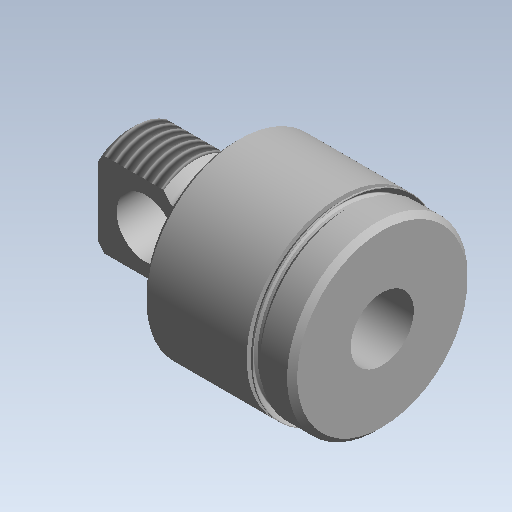
# Autodesk Inventor part: 09P0Y000_rear_head
Saved by Autodesk Inventor 2020 (Build 240168000, 168)
## iProperties
Part Number: 09P0Y000_rear_head
Material: Generic
Catalog Web Link: www.cadenas.de
Description: Rear Head-Original Line - Standard Air Cylinders
Vendor: BIMBA
Document SubType Name: Modeling
Designer: partserver
Manufacturer: BIMBA
Mass: 12.8782 g
Surface Area: 50.1592 cm^2
Volume: 12.8782 cm^3
Density: 1 g/cm^3
Appearance: PSOLRGB-211-211-211
Category: PARTsolutions
Company: BIMBA
PSOL_IDENT_0: {$CADENAS_DATA\23d-libs\bimba\bimba_brand\bimba_imperial\bimba_full_line\original_line_cylinders\sta
PSOL_IDENT_1: ndard_air_cylinders\rear_head.prj},241 {VTYP=3D},{NB=09P0Y000_rear_head},{LINA=09P0Y000_rear_head},{
PSOL_IDENT_2: NN=Rear Head},{DATE=19.01.2022 10:19:37},{GEOMDATE=11.01.2022 11:41:00},{VERSION=},{LINEID=60},{WBVA
PSOL_IDENT_3: R=MNT,ACTING,DER,Q,T1,T2,T3,T4,TRIM,Y,K,MB,CUSH,FBON},{WBNUMERIC=TRIM,MB,CUSH}  {NB=09P0Y000_rear_he
PSOL_IDENT_4: ad},{LINA=09P0Y000_rear_head},{KT=DUMMY},{PN=09P0Y000},{BORE=1.06250},{BOREPN=09},{MNT=P},{MNTALG=''
PSOL_IDENT_5: , 'Front Nose' , 'P' , 'Rear Pivot' , 'S' , 'Built-in Valve S' , 'LS' , 'Built-in Valve LS' , 'DX'
PSOL_IDENT_6: , 'Double End' , 'BR' , 'Rear Block' , 'BRT' , 'Rear Trunnion' , 'A' , 'Adjustable Stroke' , 'M' , '
PSOL_IDENT_7: Manual Valve'},{ACTING=},{ACTINGALG= '' , 'Single Acting' , 'R' , 'Reverse/Double Acting' },{DER=},{
PSOL_IDENT_8: DERALG= '' , 'Standard' },{Q=},{T1=},{T2=},{T3=},{T4=},{TRIM=0},{Y=Y},{K=},{KALG= '', 'without K', '
PSOL_IDENT_9: K', 'with K' },{MB=0},{A1=1.5000},{A1N=0.6250},{A1P=1.5000},{A1B=1.1250},{A1S=1.1250},{A2=0.25},{A2N=
PSOL_IDENT_10: 0.2500},{A3=0.0300},{D1=1.1110},{D1N=1.1155},{D1P=1.1110},{D1B=1.1410},{D2=1.0715},{C1=0.0300},{C2=0
PSOL_IDENT_11: .0300},{NDM=0.4050},{TAB=NPT},{NDMDP=0.2730},{D3=0.3440},{A4=0.1880},{A5=0.8700},{D4=0.0000},{A6=0.0
PSOL_IDENT_12: 000},{A7=0.6250},{A8=0.0000},{D5=0.0000},{D6=0.3750},{A9=0.7500},{NDM2=0.6250},{TAB2=UNF},{C11=0.030
PSOL_IDENT_13: 0},{C22=0.0000},{C33=0.0000},{C44=0.0300},{A10=0.3725},{A11=0.0000},{NDM3=0.4050},{NDM3N=0.4050},{ND
PSOL_IDENT_14: M3B=0.4050},{TAB3=NPT},{TAB3N=NPT},{TAB3B=NPT},{A12=0.594},{A12N=0.5940},{A12B=0.6880},{A13=1.2190},
PSOL_IDENT_15: {D7=0.2520},{D8=0.6225},{A14=0.0940},{A15=0.0855},{D9=0.5385},{R1=0.0350},{X1=0.0000},{X2=0.0000},{C
PSOL_IDENT_16: X=0.0000},{CC=0.0000},{CON=1},{S1=1.2500},{DB=0.2500},{X1B=0.0000},{X2B=0.0000},{A8B=0.1250},{A9B=0.
PSOL_IDENT_17: 8800},{MODEL=1},{NDM4=0.1900},{TAB4=UNF},{NDM4DP=0.3120},{BC=1.2500},{B1=0.7500},{B2=0.3800},{B3=0.5
PSOL_IDENT_18: 000},{ON=0},{ON2=1},{G1=0.3440},{G2=0.8120},{G3=0.6250},{G4=0.6245},{GD=0.2520},{G5=0.7180},{G6=0.37
PSOL_IDENT_19: 25},{RON=0},{H1=0.0000},{H2=1.1300},{H3=0.1250},{H4=0.0000},{H5=0.0000},{H6=0.0000},{F=0.5000},{PNUT=
PSOL_IDENT_20: 0.9690},{CUSH=0},{CC11=0.278},{CC111=0.2775},{CC22=0.4045},{CC33=0.2450},{CC44=0.5350},{CC55=0.7000}
PSOL_IDENT_21: ,{CD1=0.2050},{CD2=0.1360},{CD3=0.0775},{CNDM3=0.1900},{CTAB3=UNS},{OLEN=1.2190},{OD=0.3455},{STDIS=
PSOL_IDENT_22: 0.2500},{STDIS1=0.2500},{BUSHCON=D-3543},{BUSHL=0.3700},{FBON=0},{LCD=0.0000}
NB: 09P0Y000_rear_head
NN: Rear Head
NT: Original Line - Standard Air Cylinders
NBSYN: $PN._rear_head
LINA: 09P0Y000_rear_head
CATALOG: Bimba Products
PN: 09P0Y000
BORE: 1.0625
BOREPN: 09
MNT: Rear Pivot
MNTALG: '' , 'Front Nose' , 'P' , 'Rear Pivot' , 'S' , 'Built-in Valve S' , 'LS' , 'Built-in Valve LS' , 'DX' , 'Double End' , 'BR' , 'Rear Block' , 'BRT' , 'Rear Trunnion' , 'A' , 'Adjustable Stroke' , 'M' , 'Manual Valve'
ACTING: Single Acting
DER: Standard
Q: Without Side Ported Rear Head
T1: without T1
T2: without T2
T3: without T3
T4: without T4
TRIM: 0
Y: with Pivot Bushing
K: without K
MB: 0
A1N: 0.625
A1P: 1.5
A1B: 1.125
A1S: 1.125
A2N: 0.25
A3: 0.03
D1N: 1.1155
D1P: 1.111
D1B: 1.141
D2: 1.0715
C1: 0.03
C2: 0.03
TAB: NPT
NDMDP: 0.273
D3: 0.344
A4: 0.188
A5: 0.87
D4: 0
A6: 0
A7: 0.625
A8: 0
D5: 0
D6: 0.375
A9: 0.75
NDM2: 0.625
TAB2: UNF
C11: 0.03
C22: 0
C33: 0
C44: 0.03
A10: 0.3725
A11: 0
NDM3N: 0.405
NDM3B: 0.405
TAB3N: NPT
TAB3B: NPT
A12N: 0.594
A12B: 0.688
A13: 1.219
D7: 0.252
D8: 0.6225
A14: 0.094
A15: 0.0855
D9: 0.5385
R1: 0.035
X1: 0
X2: 0
CX: 0
CC: 0
S1: 1.25
DB: 0.25
X1B: 0
X2B: 0
A8B: 0.125
A9B: 0.88
NDM4: 0.19
TAB4: UNF
NDM4DP: 0.312
BC: 1.25
B1: 0.75
B2: 0.38
B3: 0.5
G1: 0.344
G2: 0.812
G3: 0.625
G4: 0.6245
GD: 0.252
G5: 0.718
G6: 0.3725
H2: 1.13
H3: 0.125
F: 0.5
CUSH: 0
CC111: 0.2775
CC22: 0.4045
CC33: 0.245
CC44: 0.535
CC55: 0.7
CD1: 0.205
CD2: 0.136
CD3: 0.0775
CNDM3: 0.19
CTAB3: UNS
OD: 0.3455
STDIS1: 0.25
BUSHCON: D-3543
BUSHL: 0.37
FBON: 0
LCD: 0
SUPPLIER: BIMBA
ARTICLENO: 09P0Y000_rear_head
BOMINFO: 09P0Y000_rear_head
CREATOR: CADENAS GmbH
Title: 09P0Y000_rear_head
Author: Cadenas PARTsolutions
Comments: Original Line - Standard Air Cylinders
Autodesk Inventor part; units mm, degrees
sketch "Sketch_18" plane through (0, 0, 0) normal (0, 0, 1) x (1, 0, 0)
  line L0 (22.225, 0) -> (0, 0)
  line L1 (0, 0) -> (0, 12.846)
  line L2 (0, 12.846) -> (0.762, 13.608)
  line L3 (0.762, 13.608) -> (4.826, 13.608)
  line L4 (4.826, 13.608) -> (5.588, 12.846)
  line L5 (5.588, 12.846) -> (6.35, 12.846)
  line L6 (6.35, 12.846) -> (6.35, 14.1097)
  line L7 (6.35, 14.1097) -> (21.463, 14.1097)
  line L8 (21.463, 14.1097) -> (22.225, 13.3477)
  line L9 (22.225, 13.3477) -> (22.225, 0)
  line L10 (22.225, 0) -> (0, 0)
  constraints: 22 end point
revolve "Revolution1" add sketch "Sketch_18" angle 360 about axis through (22.225, 0, 0) along (1, 0, 0)
sketch "Sketch_15" plane through (0, 0, 0) normal (0, 0, 1) x (1, 0, 0)
  line L0 (38.1, 0) -> (22.225, 0)
  line L1 (22.225, 0) -> (22.225, 7.9057)
  line L2 (22.225, 7.9057) -> (24.6126, 7.9057)
  line L3 (24.6126, 7.9057) -> (24.6126, 7.7279)
  arc A0 (24.6126, 7.7279) -> (25.5016, 6.839) centre (25.5016, 7.7279) ccw
  line L4 (25.5016, 6.839) -> (26.7843, 6.839)
  arc A1 (26.7843, 6.839) -> (27.383, 7.0708) centre (26.7843, 7.7279) ccw
  line L5 (27.383, 7.0708) -> (27.4129, 7.098)
  line L6 (27.4129, 7.098) -> (28.2524, 7.9375)
  line L7 (28.2524, 7.9375) -> (37.2605, 7.9375)
  line L8 (37.2605, 7.9375) -> (38.1, 7.098)
  line L9 (38.1, 7.098) -> (38.1, 0)
  line L10 (38.1, 0) -> (22.225, 0)
  constraints: 22 end point, 4 point on circle, 2 centre point
revolve "Revolution2" add sketch "Sketch_15" angle 360 about axis through (38.1, 0, 0) along (1, 0, 0)
thread "Thread1" size "5/8-18 UNF" class "2A" standard "ANSI Unified Screw Threads" full length
sketch "Sketch_70" plane through (38.1, 0, 0) normal (1, 0, 0) x (0, 0, -1)
  line L0 (-56.4388, -28.2194) -> (56.4388, -28.2194)
  line L1 (56.4388, -28.2194) -> (56.4388, 28.2194)
  line L2 (56.4388, 28.2194) -> (-56.4388, 28.2194)
  line L3 (-56.4388, 28.2194) -> (-56.4388, -28.2194)
  line L4 (-28.2194, -4.7308) -> (28.2194, -4.7308)
  line L5 (28.2194, -4.7308) -> (28.2194, 4.7308)
  line L6 (28.2194, 4.7308) -> (-28.2194, 4.7308)
  line L7 (-28.2194, 4.7308) -> (-28.2194, -4.7308)
  constraints: 16 end point
extrude "Extrusion1" cut sketch "Sketch_70" against normal blind 15.875
sketch "Sketch4" plane through (0, 0, 0) normal (-1, 0, 0) x (0, 0, 1)
  point P0 (0, 0)
hole "Hole1" at (0, 0, 0) direction (1, 0, 0) diameter 9.525 depth 20.955 tip angle 120
sketch "Sketch_47" plane through (0, 0, 0) normal (0, 0, 1) x (1, 0, 0)
  line L0 (15.0876, 0) -> (15.0876, 14.1097)
  line L1 (15.0876, 14.1097) -> (20.5423, 14.1097)
  line L2 (20.5423, 14.1097) -> (19.9073, 13.4747)
  line L3 (19.9073, 13.4747) -> (19.6754, 6.0491)
  line L4 (19.6754, 6.0491) -> (19.6754, 0)
  line L5 (19.6754, 0) -> (15.0876, 0)
  line L6 (15.0876, 0) -> (15.0876, 14.1097)
  constraints: 14 end point
revolve "Revolution3" cut sketch "Sketch_47" angle 360 about axis through (15.0876, 0, 0) along (0, -1, 0)
thread "Thread2" size "1/8" designation "1/8 - 27 NPT" standard "NPT" length 6.3023
sketch "Sketch_24" plane through (0, 0, 0) normal (0, 0, 1) x (1, 0, 0)
  line L0 (6.35, 0) -> (5.588, 0)
  line L1 (5.4861, 14.1097) -> (5.4861, 14.0255)
  line L2 (5.4861, 14.0255) -> (6.2275, 13.2842)
  arc A0 (6.2275, 13.1046) -> (6.2275, 13.2842) centre (6.1377, 13.1944) ccw
  line L3 (6.2275, 13.1046) -> (5.969, 12.846)
  line L4 (5.969, 12.846) -> (5.588, 12.846)
  line L5 (5.588, 12.846) -> (5.588, 12.5921)
  line L6 (5.588, 12.5921) -> (6.35, 12.5921)
  line L7 (6.35, 12.5921) -> (6.35, 13.449)
  line L8 (6.35, 13.449) -> (5.6893, 14.1097)
  line L9 (5.6893, 14.1097) -> (5.4861, 14.1097)
  constraints: 20 end point, 2 point on circle, 1 centre point
revolve "Revolution4" add sketch "Sketch_24" angle 360 about axis through (6.35, 0, 0) along (1, 0, 0)
sketch "Sketch_43" plane through (0, 0, 0) normal (0, 1, 0) x (-1, 0, 0)
  circle A0 centre (-30.9626, 0) radius 4.3878
  constraints: 1 centre point
extrude "Extrusion2" cut sketch "Sketch_43" along normal mid plane 14.1922
ref_plane "1_XY" through (24.6126, 0, 0) normal (1, 0, 0) x (0, 0, -1)
ref_plane "1_YZ" through (24.6126, 0, 0) normal (0, 0, -1) x (0, 1, 0)
ref_plane "1_ZX" through (24.6126, 0, 0) normal (0, 1, 0) x (1, 0, 0)
ref_plane "c1_XY" through (22.225, 7.9057, 0) normal (0, 0, 1) x (1, 0, 0)
ref_plane "c1_YZ" through (22.225, 7.9057, 0) normal (1, 0, 0) x (0, 1, 0)
ref_plane "c1_ZX" through (22.225, 7.9057, 0) normal (0, 1, 0) x (0, 0, 1)
ref_plane "c2_XY" through (22.225, -7.9057, 0) normal (0, 0, 1) x (1, 0, 0)
ref_plane "c2_YZ" through (22.225, -7.9057, 0) normal (1, 0, 0) x (0, 1, 0)
ref_plane "c2_ZX" through (22.225, -7.9057, 0) normal (0, 1, 0) x (0, 0, 1)
ref_plane "cc1_XY" through (22.225, 0, 0) normal (0, 0, 1) x (1, 0, 0)
ref_plane "cc1_YZ" through (22.225, 0, 0) normal (1, 0, 0) x (0, 1, 0)
ref_plane "cc1_ZX" through (22.225, 0, 0) normal (0, 1, 0) x (0, 0, 1)
ref_plane "cc2_XY" through (24.6126, 0, 0) normal (0, 0, 1) x (1, 0, 0)
ref_plane "cc2_YZ" through (24.6126, 0, 0) normal (1, 0, 0) x (0, 1, 0)
ref_plane "cc2_ZX" through (24.6126, 0, 0) normal (0, 1, 0) x (0, 0, 1)
ref_plane "lovra1_XY" through (33.3248, 0, 0) normal (1, 0, 0) x (0, 0, -1)
ref_plane "lovra1_YZ" through (33.3248, 0, 0) normal (0, 0, -1) x (0, 1, 0)
ref_plane "lovra1_ZX" through (33.3248, 0, 0) normal (0, 1, 0) x (1, 0, 0)
ref_plane "lovra2_XY" through (33.3248, 11.049, 0) normal (1, 0, 0) x (0, 0, -1)
ref_plane "lovra2_YZ" through (33.3248, 11.049, 0) normal (0, 0, -1) x (0, 1, 0)
ref_plane "lovra2_ZX" through (33.3248, 11.049, 0) normal (0, 1, 0) x (1, 0, 0)
ref_plane "lovra21_XY" through (0, 0, 5.2705) normal (1, 0, 0) x (0, 0, -1)
ref_plane "lovra21_YZ" through (0, 0, 5.2705) normal (0, 0, -1) x (0, 1, 0)
ref_plane "lovra21_ZX" through (0, 0, 5.2705) normal (0, 1, 0) x (1, 0, 0)
ref_plane "lovra22_XY" through (0, 0, -5.2705) normal (1, 0, 0) x (0, 0, -1)
ref_plane "lovra22_YZ" through (0, 0, -5.2705) normal (0, 0, -1) x (0, 1, 0)
ref_plane "lovra22_ZX" through (0, 0, -5.2705) normal (0, 1, 0) x (1, 0, 0)
ref_plane "lovra3_XY" through (33.3248, -11.049, 0) normal (1, 0, 0) x (0, 0, -1)
ref_plane "lovra3_YZ" through (33.3248, -11.049, 0) normal (0, 0, -1) x (0, 1, 0)
ref_plane "lovra3_ZX" through (33.3248, -11.049, 0) normal (0, 1, 0) x (1, 0, 0)
ref_plane "olen_XY" through (30.9626, 0, 0) normal (1, 0, 0) x (0, 0, -1)
ref_plane "olen_YZ" through (30.9626, 0, 0) normal (0, 0, -1) x (0, 1, 0)
ref_plane "olen_ZX" through (30.9626, 0, 0) normal (0, 1, 0) x (1, 0, 0)
ref_plane "p1_XY" through (38.1, 0, 4.7308) normal (1, 0, 0) x (0, 0, -1)
ref_plane "p1_YZ" through (38.1, 0, 4.7308) normal (0, 0, -1) x (0, 1, 0)
ref_plane "p1_ZX" through (38.1, 0, 4.7308) normal (0, 1, 0) x (1, 0, 0)
ref_plane "p2_XY" through (38.1, 0, -4.7308) normal (1, 0, 0) x (0, 0, -1)
ref_plane "p2_YZ" through (38.1, 0, -4.7308) normal (0, 0, -1) x (0, 1, 0)
ref_plane "p2_ZX" through (38.1, 0, -4.7308) normal (0, 1, 0) x (1, 0, 0)
ref_plane "port_XY" through (15.0876, 0, 0) normal (0, 0, 1) x (1, 0, 0)
ref_plane "port_YZ" through (15.0876, 0, 0) normal (1, 0, 0) x (0, 1, 0)
ref_plane "port_ZX" through (15.0876, 0, 0) normal (0, 1, 0) x (0, 0, 1)
ref_plane "port2_XY" through (38.1, 0, 0) normal (1, 0, 0) x (0, 0, -1)
ref_plane "port2_YZ" through (38.1, 0, 0) normal (0, 0, -1) x (0, 1, 0)
ref_plane "port2_ZX" through (38.1, 0, 0) normal (0, 1, 0) x (1, 0, 0)
ref_plane "thd1_XY" through (38.1, 0, 7.9375) normal (1, 0, 0) x (0, 0, -1)
ref_plane "thd1_YZ" through (38.1, 0, 7.9375) normal (0, 0, -1) x (0, 1, 0)
ref_plane "thd1_ZX" through (38.1, 0, 7.9375) normal (0, 1, 0) x (1, 0, 0)
ref_plane "thd2_XY" through (38.1, 0, -7.9375) normal (1, 0, 0) x (0, 0, -1)
ref_plane "thd2_YZ" through (38.1, 0, -7.9375) normal (0, 0, -1) x (0, 1, 0)
ref_plane "thd2_ZX" through (38.1, 0, -7.9375) normal (0, 1, 0) x (1, 0, 0)
ref_plane "to_mounting_bracket_XY" through (22.225, 0, 0) normal (1, 0, 0) x (0, 0, -1)
ref_plane "to_mounting_bracket_YZ" through (22.225, 0, 0) normal (0, 0, -1) x (0, 1, 0)
ref_plane "to_mounting_bracket_ZX" through (22.225, 0, 0) normal (0, 1, 0) x (1, 0, 0)
ref_plane "to_nut_XY" through (24.6126, 0, 0) normal (1, 0, 0) x (0, 0, -1)
ref_plane "to_nut_YZ" through (24.6126, 0, 0) normal (0, 0, -1) x (0, 1, 0)
ref_plane "to_nut_ZX" through (24.6126, 0, 0) normal (0, 1, 0) x (1, 0, 0)
ref_plane "to_pin_XY" through (30.9626, 0, 0) normal (0, 1, 0) x (1, 0, 0)
ref_plane "to_pin_YZ" through (30.9626, 0, 0) normal (1, 0, 0) x (0, 0, -1)
ref_plane "to_pin_ZX" through (30.9626, 0, 0) normal (0, 0, -1) x (0, 1, 0)
ref_plane "to_pin_1_XY" through (30.9626, 0, 0) normal (0, 0, 1) x (1, 0, 0)
ref_plane "to_pin_1_YZ" through (30.9626, 0, 0) normal (1, 0, 0) x (0, 1, 0)
ref_plane "to_pin_1_ZX" through (30.9626, 0, 0) normal (0, 1, 0) x (0, 0, 1)
ref_plane "to_pin_r_XY" through (30.9626, 0, 0) normal (0, 0, 1) x (1, 0, 0)
ref_plane "to_pin_r_YZ" through (30.9626, 0, 0) normal (1, 0, 0) x (0, 1, 0)
ref_plane "to_pin_r_ZX" through (30.9626, 0, 0) normal (0, 1, 0) x (0, 0, 1)
ref_plane "to_screw_XY" through (15.0876, 10.2743, -7.0612) normal (0, 1, 0) x (1, 0, 0)
ref_plane "to_screw_YZ" through (15.0876, 10.2743, -7.0612) normal (1, 0, 0) x (0, 0, -1)
ref_plane "to_screw_ZX" through (15.0876, 10.2743, -7.0612) normal (0, 0, -1) x (0, 1, 0)
ref_plane "to_tube_XY" through (5.588, 0, 0) normal (1, 0, 0) x (0, 0, -1)
ref_plane "to_tube_YZ" through (5.588, 0, 0) normal (0, 0, -1) x (0, 1, 0)
ref_plane "to_tube_ZX" through (5.588, 0, 0) normal (0, 1, 0) x (1, 0, 0)
body "Solid1"
